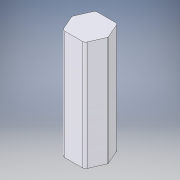
# Autodesk Inventor part: Powerbank
Saved by Autodesk Inventor 2018 (Build 220112000, 112)
## iProperties
Created: 2018-10-24
Part Number: Powerbank
Material: Generic
Document SubType Name: Modeling
Designer: iki
Density: 1 g/cm^3
Appearance: Default
Author: iki
Autodesk Inventor part; units mm, degrees
ref_plane "YZ Plane" through (0, 0, 0) normal (1, 0, 0) x (0, 1, 0)
ref_plane "XZ Plane" through (0, 0, 0) normal (0, 1, 0) x (-1, 0, 0)
ref_plane "XY Plane" through (0, 0, 0) normal (0, 0, 1) x (1, 0, 0)
sketch "Sketch1" plane through (0, 0, 0) normal (0, 0, 1) x (1, 0, 0)
  line L0 (-16.5, -15) -> (16.5, -15)
  line L1 (16.5, -15) -> (16.5, 15)
  line L2 (16.5, 15) -> (-16.5, 15)
  line L3 (-16.5, 15) -> (-16.5, -15)
  line L4 (-16.5, -15) -> (16.5, 15) construction
  line L5 (16.5, -15) -> (-16.5, 15) construction
  point P0 (0, 0)
  dimension "d0" = 33
  dimension "d1" = 30
  constraints: 12 end point, 2 midpoint, 2 parallel, 1 horizontal, 1 perpendicular
  measures "d0" distance of L2.end L1.end
  measures "d1" distance of L1.end L0.end
extrude "Extrusion1" add sketch "Sketch1" along normal mid plane 100
sketch "Sketch2" plane through (0, 0, 50) normal (0, 0, 1) x (1, 0, 0)
  line L0 (10.7831, 13.1928) -> (16.3277, 0.3976)
  arc A0 (10.7831, 13.1928) -> (8.0304, 15) centre (8.0304, 12) ccw
  line L1 (8.0304, 15) -> (16.5, 15)
  line L2 (16.5, 15) -> (16.5, 0)
  line L3 (-10.7831, 13.1928) -> (-16.3277, 0.3976)
  arc A1 (-8.0304, 15) -> (-10.7831, 13.1928) centre (-8.0304, 12) ccw
  line L4 (-8.0304, 15) -> (-16.5, 15)
  line L5 (-16.5, 15) -> (-16.5, 0)
  line L6 (10.7831, -13.1928) -> (16.3277, -0.3976)
  arc A2 (8.0304, -15) -> (10.7831, -13.1928) centre (8.0304, -12) ccw
  line L7 (8.0304, -15) -> (16.5, -15)
  line L8 (16.5, -15) -> (16.5, 0)
  line L9 (-10.7831, -13.1928) -> (-16.3277, -0.3976)
  arc A3 (-10.7831, -13.1928) -> (-8.0304, -15) centre (-8.0304, -12) ccw
  line L10 (-8.0304, -15) -> (-16.5, -15)
  line L11 (-16.5, -15) -> (-16.5, 0)
  arc A4 (-16.3277, 0.3976) -> (-16.3277, -0.3976) centre (-15.4101, 0) ccw
  arc A5 (16.3277, -0.3976) -> (16.3277, 0.3976) centre (15.4101, 0) ccw
  point P0 (0, 0)
  point P1 (10, 15)
  point P2 (-10, 15)
  point P3 (10, -15)
  point P4 (-10, -15)
  dimension "d10" = 3
  dimension "d11" = 1
  constraints: 24 end point, 12 point on circle, 8 point on line, 6 centre point, 5 tangent, 1 equal radius, 1 perpendicular
  measures "d10" radius of A0
  measures "d11" radius of A4
extrude "Extrusion2" cut sketch "Sketch2" against normal blind 100
body "Solid1"
